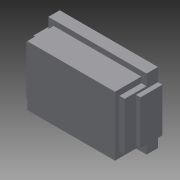
# Autodesk Inventor part: leroy_merlin_boite
Saved by Autodesk Inventor 2014 SP1 (Build 180222100, 222)
## iProperties
Created: 2015-08-04
Part Number: leroy_merlin_boite
Material: Générique
Document SubType Name: Modeling
Designer: astralien3000
Density: 1 g/cm^3
Appearance: Par défaut
Author: astralien3000
Autodesk Inventor part; units mm, degrees
ref_plane "YZ Plane" through (0, 0, 0) normal (1, 0, 0) x (0, 1, 0)
ref_plane "XZ Plane" through (0, 0, 0) normal (0, 1, 0) x (-1, 0, 0)
ref_plane "XY Plane" through (0, 0, 0) normal (0, 0, 1) x (1, 0, 0)
sketch "Esquisse1" plane through (0, 0, 0) normal (0, 1, 0) x (-1, 0, 0)
  line L0 (-50, 34) -> (50, 34)
  line L1 (50, 34) -> (50, -34)
  line L2 (50, -34) -> (-50, -34)
  line L3 (-50, -34) -> (-50, 34)
  point P0 (0, 0)
  dimension "d0" = 100
  dimension "d1" = 68
  dimension "d2" = 34
  dimension "d3" = 50
  constraints: 8 end point, 2 parallel, 1 horizontal, 1 perpendicular
  measures "d0" distance of L0.start L0.end
  measures "d1" distance of L2.end L0.start
  measures "d2" distance from line of point (0, 0) L0
  measures "d3" distance from line of L1 point (0, 0)
extrude "Extrusion1" add sketch "Esquisse1" along normal blind 30
sketch "Esquisse2" plane through (0, 30, 0) normal (0, 1, 0) x (1, 0, 0)
  line L0 (-56, 40) -> (56, 40)
  line L1 (56, 40) -> (56, -40)
  line L2 (56, -40) -> (-56, -40)
  line L3 (-56, -40) -> (-56, 40)
  point P0 (0, 0)
  dimension "d6" = 112
  dimension "d7" = 80
  dimension "d8" = 40
  dimension "d9" = 56
  constraints: 8 end point, 2 parallel, 1 horizontal, 1 perpendicular
  measures "d6" distance of L0.start L0.end
  measures "d7" distance of L2.end L0.start
  measures "d8" distance from line of point (0, 0) L0
  measures "d9" distance from line of point (0, 0) L1
extrude "Extrusion2" add sketch "Esquisse2" along normal blind 13
sketch "Esquisse3" plane through (50, 0, 34) normal (1, 0, 0) x (0, 0, -1)
  line L0 (0, 30) -> (68, 30) projected
  line L1 (6.5, 30) -> (61.5, 30)
  line L2 (61.5, 30) -> (61.5, 5)
  line L3 (61.5, 5) -> (6.5, 5)
  line L4 (6.5, 5) -> (6.5, 30)
  point P0 (34, 0)
  dimension "d12" = 25
  dimension "d13" = 55
  dimension "d14" = 27.5
  constraints: 8 end point, 2 parallel, 1 horizontal, 1 perpendicular, 1 point on line
  measures "d12" distance of L3.end L1.start
  measures "d13" distance of L2.end L3.end
  measures "d14" distance from line of point (34, 0) L2
extrude "Extrusion3" add sketch "Esquisse3" along normal up to surface (6 mm away)
sketch "Esquisse4" plane through (56, 30, -40) normal (1, 0, 0) x (0, 0, -1)
  line L0 (-80, 13) -> (0, 13) projected
  line L1 (-65, 13) -> (-15, 13)
  line L2 (-15, 13) -> (-15, -12)
  line L3 (-15, -12) -> (-65, -12)
  line L4 (-65, -12) -> (-65, 13)
  point P0 (-40, -30)
  dimension "d17" = 50
  dimension "d18" = 25
  dimension "d19" = 25
  constraints: 8 end point, 2 parallel, 1 horizontal, 1 perpendicular, 1 point on line
  measures "d17" distance of L2.end L3.end
  measures "d18" distance of L3.end L1.start
  measures "d19" distance from line of L2 point (-40, -30)
extrude "Extrusion4" add sketch "Esquisse4" along normal blind 5
mirror "Symétrie1" about plane through (0, 0, 0) normal (1, 0, 0) of "Extrusion4", "Extrusion3"
equation "\"d2\" = 0.5 * d1"
equation "\"d3\" = 0.5 * d0"
equation "\"d8\" = 0.5 * d7"
equation "\"d9\" = 0.5 * d6"
equation "\"d14\" = 0.5 * d13"
equation "\"d19\" = 0.5 * d17"
